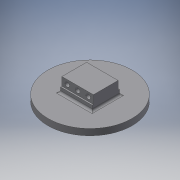
# Autodesk Inventor part: cycloid_fixing_base
Saved by Autodesk Inventor 2019.4 (Build 234330000, 330)
## iProperties
Created: 2019-09-10
Part Number: cycloid_fixing_base
Material: Generic
Document SubType Name: Modeling
Designer: cdi
Density: 1 g/cm^3
Appearance: Default
Author: cdi
Autodesk Inventor part; units mm, degrees
ref_plane "YZ Plane" through (0, 0, 0) normal (1, 0, 0) x (0, 1, 0)
ref_plane "XZ Plane" through (0, 0, 0) normal (0, 1, 0) x (-1, 0, 0)
ref_plane "XY Plane" through (0, 0, 0) normal (0, 0, 1) x (1, 0, 0)
sketch "Sketch1" plane through (0, 0, 0) normal (0, 1, 0) x (-1, 0, 0)
  line L0 (-15, 11.75) -> (-15, -11.75)
  line L1 (-15, -11.75) -> (15, -11.75)
  line L2 (15, -11.75) -> (15, 11.75)
  line L3 (15, 11.75) -> (-15, 11.75)
  line L4 (-15, 11.75) -> (15, -11.75) construction
  line L5 (-15, -11.75) -> (15, 11.75) construction
  point P0 (0, 0)
  dimension "d0" = 23.5
  dimension "d1" = 30
  constraints: 12 end point, 2 midpoint, 2 parallel, 1 perpendicular, 1 vertical
  measures "d0" distance of L1.end L2.end
  measures "d1" distance of L0.end L1.end
extrude "Extrusion1" add sketch "Sketch1" along normal blind 8
sketch "Sketch2" plane through (-15, 0, 11.75) normal (0, 0, 1) x (1, 0, 0)
  circle A0 centre (15, 4) radius 1.5
  line L0 (0, 8) -> (30, 8) projected
  point P0 (15, 0)
  dimension "d4" = 3
  dimension "d5" = 8
  dimension "d6" = 4
  constraints: 1 centre point
  measures "d4" diameter of A0
  measures "d5" distance from line of point (15, 0) L0
  measures "d6" distance of point (15, 0) A0.centre
hole "Hole1" at (0, 4, 11.75) direction (0, 0, -1) diameter 3.88 depth 7 countersink diameter 4.34 countersink angle 7
pattern_linear "Rectangular Pattern1" count 2 spacing 10 along (1, 0, 0) count 2 spacing 10 along (-1, 0, 0) of "Hole1"
mirror "Mirror1" about plane through (0, 0, 0) normal (0, 0, 1) of "Hole1", "Rectangular Pattern1"
sketch "Sketch3" plane through (0, 0, 0) normal (0, -1, 0) x (1, 0, 0)
  line L0 (-15, -13) -> (-15, 13)
  line L1 (-15, 13) -> (15, 13)
  line L2 (15, 13) -> (15, -13)
  line L3 (15, -13) -> (-15, -13)
  line L4 (-15, -13) -> (15, 13) construction
  line L5 (-15, 13) -> (15, -13) construction
  point P0 (0, 0)
  dimension "d20" = 26
  dimension "d21" = 30
  constraints: 12 end point, 2 midpoint, 2 parallel, 1 perpendicular, 1 vertical
  measures "d20" distance of L1.end L2.end
  measures "d21" distance of L0.end L1.end
extrude "Extrusion2" add sketch "Sketch3" along normal blind 5
sketch "Sketch4" plane through (0, -5, 0) normal (0, -1, 0) x (1, 0, 0)
  circle A0 centre (0, 0) radius 40
  dimension "d24" = 80
  constraints: 1 centre point, 1 coincident
  measures "d24" diameter of A0
extrude "Extrusion3" add sketch "Sketch4" along normal blind 6
fillet "Fillet1" radius 2 4 edges at (0, -5, 13) (15, -5, 0) (0, -5, -13) (-15, -5, 0)
equation "\"d6\" = 0.5 * d5"
body "Solid1"
